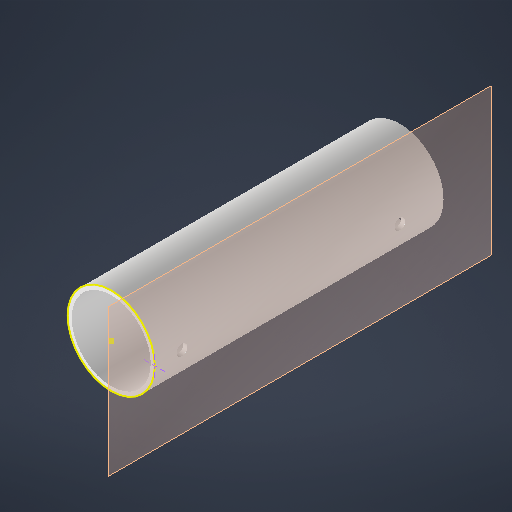
# Autodesk Inventor part: Solenoid Yoke
Saved by Autodesk Inventor 2026.3 (Build 303398000, 398)
## iProperties
Created: 2026-07-22
Part Number: Solenoid Yoke
Material: Generic
Document SubType Name: Sheet Metal
Designer: matot
Density: 1 g/cm^3
Sheet Metal Rule: Default_mm
Appearance: Default
Author: matot
Autodesk Inventor part; units mm, degrees
ref_plane "YZ Plane" through (0, 0, 0) normal (1, 0, 0) x (0, 1, 0)
ref_plane "XZ Plane" through (0, 0, 0) normal (0, 1, 0) x (-1, 0, 0)
ref_plane "XY Plane" through (0, 0, 0) normal (0, 0, 1) x (1, 0, 0)
sketch "Sketch1" plane through (0, 0, 0) normal (0, 0, 1) x (1, 0, 0)
  circle A0 centre (0, 0) radius 14.5
  circle A1 centre (0, 0) radius 16
  dimension "d0" = 29
  dimension "d1" = 32
  constraints: 2 centre point, 2 coincident
  measures "d0" diameter of A0
  measures "d1" diameter of A1
extrude "Extrusion1" add sketch "Sketch1" along normal blind 106
sketch "Sketch4" plane through (0, 0, 106) normal (0, 0, 1) x (1, 0, 0)
  circle A0 centre (0, 0) radius 16 projected
  point P0 (16, 0)
  constraints: 1 horizontal alignment, 1 other
ref_plane "Work Plane1" through (16, 0, 106) normal (1, 0, 0) x (0, 1, 0)
sketch "Sketch5" plane through (16, 0, 106) normal (1, 0, 0) x (0, 1, 0)
  line L0 (16, 0) -> (-16, 0) projected
  point P0 (0, -106)
  point P1 (0, -10)
  point P2 (0, -90)
  dimension "d11" = 10
  dimension "d12" = 80
  measures "d11" distance from line of point (0, -10) L0
  measures "d12" distance of point (0, -90) point (0, -10)
hole "Hole1" at (16, 0, 96) at (16, 0, 16) direction (-1, 0, 0) diameter 4 depth 5 tip angle 118
equation "\"BendRadius\" = Thickness"
equation "\"BendReliefWidth\" = Thickness"
equation "\"BendReliefDepth\" = 0.5 * Thickness"
equation "\"CornerReliefSize\" = 4 * Thickness"
equation "\"MinimumRemnant\" = 2 * Thickness"
equation "\"TransitionRadius\" = BendRadius"
equation "\"JacobiRadiusSize\" = BendRadius"
equation "\"GapSize\" = Thickness"
equation "\"Thickness\" = 0.5"
body "Solid1"
